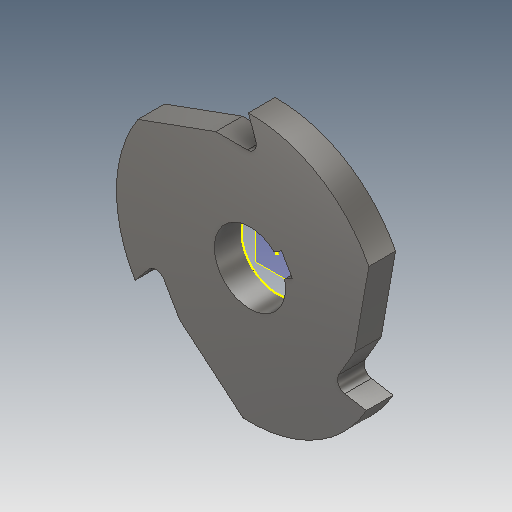
# Autodesk Inventor part: pisau ok2
Saved by Autodesk Inventor 2017 (Build 210142000, 142)
## iProperties
Created: 2017-08-25
Part Number: pisau ok2
Material: Stainless Steel
Document SubType Name: Modeling
Designer: Sigit
Density: 8 g/cm^3
Appearance: Semi-Polished
Mass: 1640.9 g
Surface Area: 370.096 cm^2
Volume: 205.113 cm^3
Author: Sigit
Autodesk Inventor part; units mm, degrees
ref_plane "YZ Plane" through (0, 0, 0) normal (1, 0, 0) x (0, 1, 0)
ref_plane "XZ Plane" through (0, 0, 0) normal (0, 1, 0) x (-1, 0, 0)
ref_plane "XY Plane" through (0, 0, 0) normal (0, 0, 1) x (1, 0, 0)
sketch "Sketch1" plane through (0, 0, 0) normal (0, 0, 1) x (1, 0, 0)
  line L0 (-74.9186, 47.1822) -> (53.4099, 57.2393) construction
  line L1 (53.4099, 57.2393) -> (63.1167, -66.6187) construction
  line L2 (63.1167, -66.6187) -> (-65.2118, -76.6758) construction
  line L3 (-65.2118, -76.6758) -> (-74.9186, 47.1822) construction
  line L4 (6, 16) -> (-6, 24) construction
  line L5 (0, 20) -> (6, 24) construction
  circle A0 centre (1.0672, -0.4938) radius 75
  line L6 (1.0672, 74.5062) -> (1.0672, -0.4938) construction
  line L7 (1.0672, 74.5062) -> (5.6579, 61.8933)
  line L8 (1.0672, 74.5062) -> (14.4896, 74.5062) construction
  line L9 (1.3501, 55.1985) -> (-17.016, 53.7591)
  line L10 (-17.016, 53.7591) -> (-67, 31)
  arc A1 (1.3501, 55.1985) -> (5.6579, 61.8933) centre (0.9595, 60.1832) ccw
  circle A2 centre (1.0672, -0.4938) radius 20
  point P0 (0, 0)
  point P1 (7.9076, 55.7124)
  dimension "d2" = 12
  dimension "d4" = 150
  dimension "d5" = 20
  dimension "d6" = 70
  dimension "d8" = 25
  dimension "d10" = 160
  dimension "d11" = 5
  dimension "d23" = 40
  constraints: 14 end point, 4 point on circle, 3 centre point, 2 point on line, 2 tangent, 1 coincident, 1 equal length, 1 horizontal, 1 midpoint, 1 parallel, 1 vertical, 2 other
  measures "d2" distance of L4.end L5.end
  measures "d4" diameter of A0
  measures "d5" distance of L6.start point (7.908, 55.712)
  measures "d6" angle of L7 L8
  measures "d8" distance of point (7.908, 55.712) L9.end
  measures "d10" angle of L10 L9
  measures "d11" radius of A1
  measures "d23" diameter of A2
ref_plane "Work Plane1" through (0, 0, 0) normal (0, 0, -1) x (-1, 0, 0)
sketch "Sketch2" plane through (0, 0, 0) normal (0, 0, -1) x (-1, 0, 0)
  line L0 (0, 75) -> (-4.3981, 62.9162) projected
  arc A0 (-4.3981, 62.9162) -> (0.3003, 56.2061) centre (0.3003, 61.2061) ccw projected
  line L1 (0.3003, 56.2061) -> (18.1596, 56.2061) projected
  line L2 (18.1596, 56.2061) -> (63.6666, 39.643) projected
  arc A1 (63.6666, 39.643) -> (0, 75) centre (27.2068, 48.9906) ccw
  point P0 (0, 0)
  constraints: 2 point on circle, 1 centre point
extrude "Extrusion3" add sketch "Sketch1" along normal blind 15
extrude "Extrusion4" cut sketch "Sketch2" against normal blind 15
pattern_circular "Circular Pattern2" count 3 over 360 about axis through (1.0672, -0.4938, 0) along (0, 0, 1) of "Extrusion4"
sketch "Sketch3" plane through (0, 0, 0) normal (0, 0, -1) x (-1, 0, 0)
  circle A0 centre (-1.0672, -0.4938) radius 20 projected
  point P0 (0, 0)
sketch "Sketch4" plane through (0, 0, 15) normal (0, 0, 1) x (1, 0, 0)
  circle A0 centre (1.0672, -0.4938) radius 20 projected
  line L0 (17.9236, 2.3101) -> (11.9236, 12.7024)
  line L1 (11.9236, 12.7024) -> (18.8518, 16.7024)
  line L2 (18.8518, 16.7024) -> (24.8518, 6.3101)
  line L3 (24.8518, 6.3101) -> (17.9236, 2.3101)
  line L4 (17.9236, 2.3101) -> (18.8518, 16.7024) construction
  line L5 (11.9236, 12.7024) -> (24.8518, 6.3101) construction
  point P0 (0, 0)
  point P1 (18.3877, 9.5062)
  dimension "d35" = 12
  dimension "d36" = 8
  constraints: 12 end point, 2 midpoint, 2 parallel, 1 perpendicular, 2 other
  measures "d35" distance of L1.end L2.end
  measures "d36" distance of L0.end L1.end
extrude "Extrusion5" cut sketch "Sketch4" against normal through all contours L3 L0 L1 A0 | A0 L1 L2 L3 picked at (15.7106, 8.7411)
body "Solid1"
